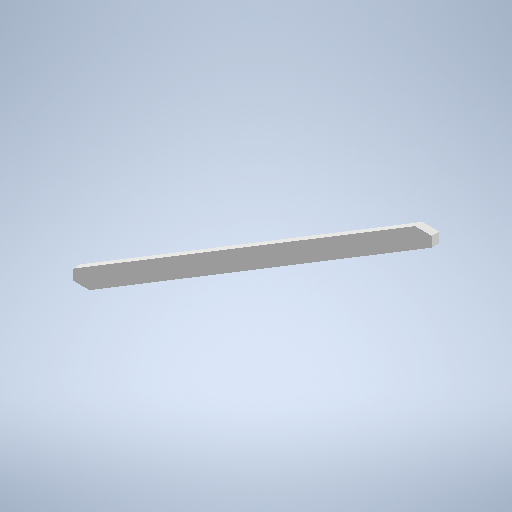
# Autodesk Inventor part: side1
Saved by Autodesk Inventor 2025.1 (Build 291241020, 241B)
## iProperties
Created: 2024-09-16
Part Number: side1
Material: Generic
Document SubType Name: Modeling
Designer: User
Density: 1 g/cm^3
Appearance: Default
Author: User
Autodesk Inventor part; units mm, degrees
ref_plane "YZ Plane" through (0, 0, 0) normal (1, 0, 0) x (0, 1, 0)
ref_plane "XZ Plane" through (0, 0, 0) normal (0, 1, 0) x (-1, 0, 0)
ref_plane "XY Plane" through (0, 0, 0) normal (0, 0, 1) x (1, 0, 0)
sketch "Sketch1" plane through (0, 0, 0) normal (0, 0, 1) x (1, 0, 0)
  line L0 (914.4, 1200.15) -> (-914.4, 1200.15) projected
  line L1 (914.4, 0) -> (914.4, 4876.8) projected
  line L2 (-914.4, 4876.8) -> (-914.4, 0) projected
  line L3 (914.4, 88.9) -> (-914.4, 88.9) projected
  line L4 (914.4, 1148.1373) -> (-828.802, 88.9)
  line L5 (-914.4, 140.9127) -> (828.802, 1200.15)
  line L6 (-828.802, 88.9) -> (-914.4, 88.9)
  line L7 (-914.4, 88.9) -> (-914.4, 140.9127)
  line L8 (914.4, 1148.1373) -> (914.4, 1200.15)
  line L9 (914.4, 1200.15) -> (828.802, 1200.15)
  point P0 (0, 0)
  point P1 (42.799, 618.5187)
  constraints: 12 end point, 4 collinear, 4 point on line, 1 midpoint, 1 parallel, 2 other
extrude "Extrusion1" add sketch "Sketch1" against normal blind 38.1 contours L1 L4 L3 L2 L5 L0
body "Solid1"
